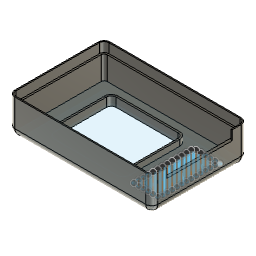
CO2_tapa_modelo (Autodesk Fusion 360 design; units mm, degrees)
Autodesk Fusion 360 part; units mm, degrees
sketch "Sketch1" plane through (0, 0, 0) normal (0, 0, 1) x (1, 0, 0)
  line L0 (55, 40) -> (-55, 40)
  line L1 (-60, 35) -> (-60, -35)
  line L2 (-55, -40) -> (55, -40)
  line L3 (60, -35) -> (60, 35)
  line L4 (60, 40) -> (-60, -40) construction
  line L5 (-60, 40) -> (60, -40) construction
  arc A0 (60, 35) -> (55, 40) centre (55, 35) ccw
  arc A1 (-55, 40) -> (-60, 35) centre (-55, 35) ccw
  arc A2 (55, -40) -> (60, -35) centre (55, -35) ccw
  arc A3 (-60, -35) -> (-55, -40) centre (-55, -35) ccw
  dimension "d1" = 120
  dimension "d2" = 80
  dimension "d3" = 5
  dimension "d4" = 5
  dimension "d5" = 5
  dimension "d6" = 5
  constraint horizontal L0
  constraint perpendicular L0 L1
  constraint parallel L0 L2
  constraint parallel L1 L3
  constraint coincident L4 origin
  constraint coincident L5 origin
  constraint coincident L4.start L0
  constraint coincident L4.start L3
  constraint tangent L0 A0
  constraint tangent L3 A0
  constraint coincident L5.start L0
  constraint coincident L5.start L1
  constraint tangent L0 A1
  constraint tangent L1 A1
  constraint coincident L5.end L3
  constraint coincident L5.end L2
  constraint tangent L3 A2
  constraint tangent L2 A2
  constraint coincident L4.end L1
  constraint coincident L4.end L2
  constraint tangent L1 A3
  constraint tangent L2 A3
  measures "d1" distance of L4.end L5.end
  measures "d2" distance of L5.start L4.end
  measures "d3" radius of A0
  measures "d4" radius of A1
  measures "d5" radius of A2
  measures "d6" radius of A3
extrude "Extrude1" add sketch "Sketch1" along normal blind 30
shell "Shell1" thickness 2.5 removed faces 1 at (18.3333, -13.3333, 30)
sketch "Sketch2" plane through (0, 0, 30) normal (0, 0, 1) x (-1, 0, 0)
  line L0 (57.5, 35) -> (57.5, -35)
  arc A0 (55, -37.5) -> (57.5, -35) centre (55, -35) ccw
  line L1 (55, -37.5) -> (-55, -37.5)
  arc A1 (-57.5, -35) -> (-55, -37.5) centre (-55, -35) ccw
  line L2 (-57.5, -35) -> (-57.5, 35)
  arc A2 (-55, 37.5) -> (-57.5, 35) centre (-55, 35) ccw
  line L3 (-55, 37.5) -> (55, 37.5)
  arc A3 (57.5, 35) -> (55, 37.5) centre (55, 35) ccw
  arc A4 (60, 35) -> (55, 40) centre (55, 35) ccw
  line L4 (55, 40) -> (-55, 40)
  arc A5 (-55, 40) -> (-60, 35) centre (-55, 35) ccw
  line L5 (-60, 35) -> (-60, -35)
  arc A6 (-60, -35) -> (-55, -40) centre (-55, -35) ccw
  line L6 (-55, -40) -> (55, -40)
  arc A7 (55, -40) -> (60, -35) centre (55, -35) ccw
  line L7 (60, -35) -> (60, 35)
  arc A8 (-59, -35) -> (-55, -39) centre (-55, -35) ccw
  line L8 (55, -39) -> (-55, -39)
  arc A9 (55, -39) -> (59, -35) centre (55, -35) ccw
  line L9 (59, 35) -> (59, -35)
  arc A10 (59, 35) -> (55, 39) centre (55, 35) ccw
  line L10 (-55, 39) -> (55, 39)
  arc A11 (-55, 39) -> (-59, 35) centre (-55, 35) ccw
  line L11 (-59, -35) -> (-59, 35)
  dimension "d10" = -1.5
extrude "Extrude2" cut sketch "Sketch2" against normal blind 8 contours A8 L8 A9 L9 A10 L10 A11 L11
sketch "Sketch3" plane through (60, 0, 0) normal (1, 0, 0) x (0, 1, 0)
  line L0 (-35, 0) -> (35, 0)
  line L1 (35, 0) -> (35, 30)
  line L2 (35, 30) -> (-35, 30)
  line L3 (-35, 30) -> (-35, 0)
  line L4 (27.5, 22) -> (-27.5, 22)
  line L5 (-27.5, 22) -> (-27.5, 38)
  line L6 (-27.5, 38) -> (27.5, 38)
  line L7 (27.5, 38) -> (27.5, 22)
  line L8 (27.5, 22) -> (-27.5, 38) construction
  line L9 (-27.5, 22) -> (27.5, 38) construction
  point P0 (0, 30)
  dimension "d13" = 55
  dimension "d14" = 16
  constraint horizontal L4
  constraint perpendicular L4 L5
  constraint parallel L4 L6
  constraint parallel L5 L7
  constraint coincident L8 P0
  constraint coincident L9 P0
  constraint midpoint L2 P0
  measures "d13" distance of L5.end L6.end
  measures "d14" distance of L4.end L5.end
extrude "Extrude3" cut sketch "Sketch3" against normal blind 25 contours L2 L5 L6 L7 | L2 L4 L5 L7
fillet "Fillet1" radius 7 1 faces at (18.3333, -13.3333, 0)
sketch "Sketch4" plane through (0, 0, 0) normal (0, 0, -1) x (1, 0, 0)
  line L0 (-53, 33) -> (-53, -33)
  line L1 (-53, -33) -> (53, -33)
  line L2 (53, -33) -> (53, 33)
  line L3 (53, 33) -> (-53, 33)
sketch "Sketch5" plane through (0, 0, 0) normal (0, 0, 1) x (1, 0, 0)
  line L0 (-59, 0) -> (-9, 0) construction
  line L1 (-9, 0) -> (-9, -45) construction
  circle A0 centre (-9, 0) radius 7 construction
  line L2 (17, -25) -> (-35, -25)
  line L3 (-39, -21) -> (-39, 21)
  line L4 (-35, 25) -> (17, 25)
  line L5 (21, 21) -> (21, -21)
  line L6 (21, -25) -> (-39, 25) construction
  line L7 (-39, -25) -> (21, 25) construction
  arc A1 (-39, -21) -> (-35, -25) centre (-35, -21) ccw
  arc A2 (17, -25) -> (21, -21) centre (17, -21) ccw
  arc A3 (-35, 25) -> (-39, 21) centre (-35, 21) ccw
  arc A4 (21, 21) -> (17, 25) centre (17, 21) ccw
  point P0 (-9, 0)
  dimension "d19" = 50
  dimension "d20" = 14
  dimension "d21" = 60
  dimension "d22" = 50
  dimension "d23" = 4
  dimension "d24" = 4
  dimension "d25" = 4
  dimension "d26" = 4
  constraint horizontal L0
  constraint perpendicular L0 L1
  constraint coincident P0 L0.end
  constraint horizontal L2
  constraint perpendicular L2 L3
  constraint parallel L2 L4
  constraint parallel L3 L5
  constraint coincident L6 P0
  constraint coincident L7 P0
  constraint coincident L7.start L2
  constraint coincident L7.start L3
  constraint tangent L2 A1
  constraint tangent L3 A1
  constraint coincident L6.start L2
  constraint coincident L6.start L5
  constraint tangent L2 A2
  constraint tangent L5 A2
  constraint coincident L6.end L3
  constraint coincident L6.end L4
  constraint tangent L3 A3
  constraint tangent L4 A3
  constraint coincident L7.end L4
  constraint coincident L7.end L5
  constraint tangent L4 A4
  constraint tangent L5 A4
  measures "d19" distance of L0.start P0
  measures "d20" diameter of A0
  measures "d21" distance of L6.end L7.end
  measures "d22" distance of L7.start L6.end
  measures "d23" radius of A1
  measures "d24" radius of A2
  measures "d25" radius of A3
  measures "d26" radius of A4
extrude "Extrude4" cut sketch "Sketch5" along normal blind 19
sketch "Sketch6" plane through (0, 0, 2.5) normal (0, 0, 1) x (-1, 0, 0)
  line L0 (-17, 25) -> (35, 25)
  arc A0 (39, 21) -> (35, 25) centre (35, 21) ccw
  line L1 (39, 21) -> (39, -21)
  arc A1 (35, -25) -> (39, -21) centre (35, -21) ccw
  line L2 (35, -25) -> (-17, -25)
  arc A2 (-21, -21) -> (-17, -25) centre (-17, -21) ccw
  line L3 (-21, -21) -> (-21, 21)
  arc A3 (-17, 25) -> (-21, 21) centre (-17, 21) ccw
  arc A4 (57.5, 35) -> (55, 37.5) centre (55, 35) ccw
  line L4 (55, 37.5) -> (-55, 37.5)
  arc A5 (-55, 37.5) -> (-57.5, 35) centre (-55, 35) ccw
  line L5 (-57.5, 35) -> (-57.5, -35)
  arc A6 (-57.5, -35) -> (-55, -37.5) centre (-55, -35) ccw
  line L6 (-55, -37.5) -> (55, -37.5)
  arc A7 (55, -37.5) -> (57.5, -35) centre (55, -35) ccw
  line L7 (57.5, -35) -> (57.5, 35)
  arc A8 (-22.5, -21) -> (-17, -26.5) centre (-17, -21) ccw
  line L8 (35, -26.5) -> (-17, -26.5)
  arc A9 (35, -26.5) -> (40.5, -21) centre (35, -21) ccw
  line L9 (40.5, 21) -> (40.5, -21)
  arc A10 (40.5, 21) -> (35, 26.5) centre (35, 21) ccw
  line L10 (-17, 26.5) -> (35, 26.5)
  arc A11 (-17, 26.5) -> (-22.5, 21) centre (-17, 21) ccw
  line L11 (-22.5, -21) -> (-22.5, 21)
  dimension "d29" = -1.5
extrude "Extrude5" add sketch "Sketch6" along normal blind 5 contours A8 L8 A9 L9 A10 L10 A11 L11
sketch "Sketch7" plane through (0, 0, 2.5) normal (0, 0, 1) x (-1, 0, 0)
  line L0 (35, -26.5) -> (-17, -26.5)
  arc A0 (-22.5, -21) -> (-17, -26.5) centre (-17, -21) ccw
  line L1 (-22.5, -21) -> (-22.5, 21)
  arc A1 (-17, 26.5) -> (-22.5, 21) centre (-17, 21) ccw
  line L2 (-17, 26.5) -> (35, 26.5)
  arc A2 (40.5, 21) -> (35, 26.5) centre (35, 21) ccw
  line L3 (40.5, 21) -> (40.5, -21)
  arc A3 (35, -26.5) -> (40.5, -21) centre (35, -21) ccw
  arc A4 (57.5, 35) -> (55, 37.5) centre (55, 35) ccw
  line L4 (55, 37.5) -> (-55, 37.5)
  arc A5 (-55, 37.5) -> (-57.5, 35) centre (-55, 35) ccw
  line L5 (-57.5, 35) -> (-57.5, -35)
  arc A6 (-57.5, -35) -> (-55, -37.5) centre (-55, -35) ccw
  line L6 (-55, -37.5) -> (55, -37.5)
  arc A7 (55, -37.5) -> (57.5, -35) centre (55, -35) ccw
  line L7 (57.5, -35) -> (57.5, 35)
  line L8 (-30, -25) -> (-51, -25) construction
  line L9 (-51, -25) -> (-51, 25) construction
  line L10 (-51, 25) -> (-30, 25) construction
  line L11 (-30, 25) -> (-30, -25) construction
  line L12 (-47.2929, -24.2929) -> (-50.2929, -21.2929)
  arc A8 (-50.2929, -21.2929) -> (-51.7071, -22.7071) centre (-51, -22) ccw
  line L13 (-51.7071, -22.7071) -> (-48.7071, -25.7071)
  arc A9 (-48.7071, -25.7071) -> (-47.2929, -24.2929) centre (-48, -25) ccw
  line L14 (-48, -25) -> (-51, -22) construction
  line L15 (-43.2929, -24.2929) -> (-50.2929, -17.2929)
  arc A10 (-50.2929, -17.2929) -> (-51.7071, -18.7071) centre (-51, -18) ccw
  line L16 (-51.7071, -18.7071) -> (-44.7071, -25.7071)
  arc A11 (-44.7071, -25.7071) -> (-43.2929, -24.2929) centre (-44, -25) ccw
  line L17 (-44, -25) -> (-51, -18) construction
  line L18 (-39.2929, -24.2929) -> (-50.2929, -13.2929)
  arc A12 (-50.2929, -13.2929) -> (-51.7071, -14.7071) centre (-51, -14) ccw
  line L19 (-51.7071, -14.7071) -> (-40.7071, -25.7071)
  arc A13 (-40.7071, -25.7071) -> (-39.2929, -24.2929) centre (-40, -25) ccw
  line L20 (-40, -25) -> (-51, -14) construction
  line L21 (-35.2929, -24.2929) -> (-50.2929, -9.2929)
  arc A14 (-50.2929, -9.2929) -> (-51.7071, -10.7071) centre (-51, -10) ccw
  line L22 (-51.7071, -10.7071) -> (-36.7071, -25.7071)
  arc A15 (-36.7071, -25.7071) -> (-35.2929, -24.2929) centre (-36, -25) ccw
  line L23 (-36, -25) -> (-51, -10) construction
  line L24 (-31.2929, -24.2929) -> (-50.2929, -5.2929)
  arc A16 (-50.2929, -5.2929) -> (-51.7071, -6.7071) centre (-51, -6) ccw
  line L25 (-51.7071, -6.7071) -> (-32.7071, -25.7071)
  arc A17 (-32.7071, -25.7071) -> (-31.2929, -24.2929) centre (-32, -25) ccw
  line L26 (-32, -25) -> (-51, -6) construction
  line L27 (-29.2929, -22.2929) -> (-50.2929, -1.2929)
  arc A18 (-50.2929, -1.2929) -> (-51.7071, -2.7071) centre (-51, -2) ccw
  line L28 (-51.7071, -2.7071) -> (-30.7071, -23.7071)
  arc A19 (-30.7071, -23.7071) -> (-29.2929, -22.2929) centre (-30, -23) ccw
  line L29 (-30, -23) -> (-51, -2) construction
  line L30 (-29.2929, -18.2929) -> (-50.2929, 2.7071)
  arc A20 (-50.2929, 2.7071) -> (-51.7071, 1.2929) centre (-51, 2) ccw
  line L31 (-51.7071, 1.2929) -> (-30.7071, -19.7071)
  arc A21 (-30.7071, -19.7071) -> (-29.2929, -18.2929) centre (-30, -19) ccw
  line L32 (-30, -19) -> (-51, 2) construction
  line L33 (-29.2929, -14.2929) -> (-50.2929, 6.7071)
  arc A22 (-50.2929, 6.7071) -> (-51.7071, 5.2929) centre (-51, 6) ccw
  line L34 (-51.7071, 5.2929) -> (-30.7071, -15.7071)
  arc A23 (-30.7071, -15.7071) -> (-29.2929, -14.2929) centre (-30, -15) ccw
  line L35 (-30, -15) -> (-51, 6) construction
  line L36 (-29.2929, -10.2929) -> (-50.2929, 10.7071)
  arc A24 (-50.2929, 10.7071) -> (-51.7071, 9.2929) centre (-51, 10) ccw
  line L37 (-51.7071, 9.2929) -> (-30.7071, -11.7071)
  arc A25 (-30.7071, -11.7071) -> (-29.2929, -10.2929) centre (-30, -11) ccw
  line L38 (-30, -11) -> (-51, 10) construction
  line L39 (-29.2929, -6.2929) -> (-50.2929, 14.7071)
  arc A26 (-50.2929, 14.7071) -> (-51.7071, 13.2929) centre (-51, 14) ccw
  line L40 (-51.7071, 13.2929) -> (-30.7071, -7.7071)
  arc A27 (-30.7071, -7.7071) -> (-29.2929, -6.2929) centre (-30, -7) ccw
  line L41 (-30, -7) -> (-51, 14) construction
  line L42 (-29.2929, -2.2929) -> (-50.2929, 18.7071)
  arc A28 (-50.2929, 18.7071) -> (-51.7071, 17.2929) centre (-51, 18) ccw
  line L43 (-51.7071, 17.2929) -> (-30.7071, -3.7071)
  arc A29 (-30.7071, -3.7071) -> (-29.2929, -2.2929) centre (-30, -3) ccw
  line L44 (-30, -3) -> (-51, 18) construction
  line L45 (-29.2929, 1.7071) -> (-50.2929, 22.7071)
  arc A30 (-50.2929, 22.7071) -> (-51.7071, 21.2929) centre (-51, 22) ccw
  line L46 (-51.7071, 21.2929) -> (-30.7071, 0.2929)
  arc A31 (-30.7071, 0.2929) -> (-29.2929, 1.7071) centre (-30, 1) ccw
  line L47 (-30, 1) -> (-51, 22) construction
  line L48 (-29.2929, 5.7071) -> (-49.2929, 25.7071)
  arc A32 (-49.2929, 25.7071) -> (-50.7071, 24.2929) centre (-50, 25) ccw
  line L49 (-50.7071, 24.2929) -> (-30.7071, 4.2929)
  arc A33 (-30.7071, 4.2929) -> (-29.2929, 5.7071) centre (-30, 5) ccw
  line L50 (-30, 5) -> (-50, 25) construction
  line L51 (-29.2929, 9.7071) -> (-45.2929, 25.7071)
  arc A34 (-45.2929, 25.7071) -> (-46.7071, 24.2929) centre (-46, 25) ccw
  line L52 (-46.7071, 24.2929) -> (-30.7071, 8.2929)
  arc A35 (-30.7071, 8.2929) -> (-29.2929, 9.7071) centre (-30, 9) ccw
  line L53 (-30, 9) -> (-46, 25) construction
  line L54 (-29.2929, 13.7071) -> (-41.2929, 25.7071)
  arc A36 (-41.2929, 25.7071) -> (-42.7071, 24.2929) centre (-42, 25) ccw
  line L55 (-42.7071, 24.2929) -> (-30.7071, 12.2929)
  arc A37 (-30.7071, 12.2929) -> (-29.2929, 13.7071) centre (-30, 13) ccw
  line L56 (-30, 13) -> (-42, 25) construction
  line L57 (-29.2929, 17.7071) -> (-37.2929, 25.7071)
  arc A38 (-37.2929, 25.7071) -> (-38.7071, 24.2929) centre (-38, 25) ccw
  line L58 (-38.7071, 24.2929) -> (-30.7071, 16.2929)
  arc A39 (-30.7071, 16.2929) -> (-29.2929, 17.7071) centre (-30, 17) ccw
  line L59 (-30, 17) -> (-38, 25) construction
  line L60 (-29.2929, 21.7071) -> (-33.2929, 25.7071)
  arc A40 (-33.2929, 25.7071) -> (-34.7071, 24.2929) centre (-34, 25) ccw
  line L61 (-34.7071, 24.2929) -> (-30.7071, 20.2929)
  arc A41 (-30.7071, 20.2929) -> (-29.2929, 21.7071) centre (-30, 21) ccw
  line L62 (-30, 21) -> (-34, 25) construction
  circle A42 centre (-30, 25) radius 1
  circle A43 centre (-52, -25) radius 1
  dimension "d32" = 2
  dimension "d33" = 2
  dimension "d34" = 2
  dimension "d35" = 2
  dimension "d36" = 2
  dimension "d37" = 2
  dimension "d38" = 2
  dimension "d39" = 2
  dimension "d40" = 2
  dimension "d41" = 2
  dimension "d42" = 2
  dimension "d43" = 2
  dimension "d44" = 2
  dimension "d45" = 2
  dimension "d46" = 2
  dimension "d47" = 2
  dimension "d48" = 2
  dimension "d49" = 2
  dimension "d48" = 2
  constraint horizontal L8
  constraint vertical L9
  constraint horizontal L10
  constraint vertical L11
  constraint tangent L12 A8
  constraint tangent A8 L13
  constraint parallel L12 L13
  constraint tangent L13 A9
  constraint tangent L12 A9
  constraint coincident L9 A8.centre
  constraint coincident L8 A9.centre
  constraint tangent L15 A10
  constraint tangent A10 L16
  constraint parallel L15 L16
  constraint tangent L16 A11
  constraint tangent L15 A11
  constraint coincident L9 A10.centre
  constraint coincident L8 A11.centre
  constraint tangent L18 A12
  constraint tangent A12 L19
  constraint parallel L18 L19
  constraint tangent L19 A13
  constraint tangent L18 A13
  constraint coincident L8 A13.centre
  constraint tangent L21 A14
  constraint tangent A14 L22
  constraint parallel L21 L22
  constraint tangent L22 A15
  constraint tangent L21 A15
  constraint coincident L9 A14.centre
  constraint coincident L8 A15.centre
  constraint tangent L24 A16
  constraint tangent A16 L25
  constraint parallel L24 L25
  constraint tangent L25 A17
  constraint tangent L24 A17
  constraint coincident L9 A16.centre
  constraint coincident L8 A17.centre
  constraint tangent L27 A18
  constraint tangent A18 L28
  constraint parallel L27 L28
  constraint tangent L28 A19
  constraint tangent L27 A19
  constraint coincident L9 A18.centre
  constraint coincident L11 A19.centre
  constraint tangent L30 A20
  constraint tangent A20 L31
  constraint parallel L30 L31
  constraint tangent L31 A21
  constraint tangent L30 A21
  constraint coincident L9 A20.centre
  constraint coincident L11 A21.centre
  constraint tangent L33 A22
  constraint tangent A22 L34
  constraint parallel L33 L34
  constraint tangent L34 A23
  constraint tangent L33 A23
  constraint coincident L9 A22.centre
  constraint parallel L30 L35
  constraint coincident L11 A23.centre
  constraint tangent L36 A24
  constraint tangent A24 L37
  constraint parallel L36 L37
  constraint tangent L37 A25
  constraint tangent L36 A25
  constraint coincident L9 A24.centre
  constraint coincident L11 A25.centre
  constraint tangent L39 A26
  constraint tangent A26 L40
  constraint parallel L39 L40
  constraint tangent L40 A27
  constraint tangent L39 A27
  constraint coincident L9 A26.centre
  constraint coincident L11 A27.centre
  constraint tangent L42 A28
  constraint tangent A28 L43
  constraint parallel L42 L43
  constraint tangent L43 A29
  constraint tangent L42 A29
  constraint coincident L9 A28.centre
  constraint parallel L39 L44
  constraint coincident L11 A29.centre
  constraint tangent L45 A30
  constraint tangent A30 L46
  constraint parallel L45 L46
  constraint tangent L46 A31
  constraint tangent L45 A31
  constraint coincident L9 A30.centre
  constraint coincident L11 A31.centre
  constraint tangent L48 A32
  constraint tangent A32 L49
  constraint parallel L48 L49
  constraint tangent L49 A33
  constraint tangent L48 A33
  constraint coincident L10 A32.centre
  constraint coincident L11 A33.centre
  constraint tangent L51 A34
  constraint tangent A34 L52
  constraint parallel L51 L52
  constraint tangent L52 A35
  constraint tangent L51 A35
  constraint coincident L10 A34.centre
  constraint coincident L11 A35.centre
  constraint tangent L54 A36
  constraint tangent A36 L55
  constraint parallel L54 L55
  constraint tangent L55 A37
  constraint tangent L54 A37
  constraint coincident L10 A36.centre
  constraint coincident L11 A37.centre
  constraint tangent L57 A38
  constraint tangent A38 L58
  constraint parallel L57 L58
  constraint tangent L58 A39
  constraint tangent L57 A39
  constraint coincident L10 A38.centre
  constraint parallel L54 L59
  constraint coincident L11 A39.centre
  constraint tangent L60 A40
  constraint tangent A40 L61
  constraint parallel L60 L61
  constraint tangent L61 A41
  constraint tangent L60 A41
  constraint coincident L10 A40.centre
  constraint coincident L11 A41.centre
  constraint coincident L10.end L11.start
  measures "d32" diameter of A8
  measures "d33" diameter of A10
  measures "d34" diameter of A12
  measures "d35" diameter of A14
  measures "d36" diameter of A16
  measures "d37" diameter of A18
  measures "d38" diameter of A20
  measures "d39" diameter of A22
  measures "d40" diameter of A24
  measures "d41" diameter of A26
  measures "d42" diameter of A28
  measures "d43" diameter of A30
  measures "d44" diameter of A32
  measures "d45" diameter of A34
  measures "d46" diameter of A36
  measures "d47" diameter of A38
  measures "d48" diameter of A40
  measures "d49" diameter of A43
